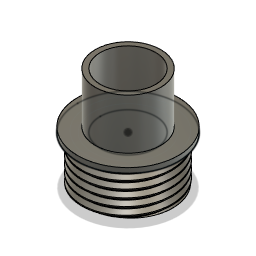
Naustok_vrch (Autodesk Fusion 360 design; units mm, degrees)
Autodesk Fusion 360 part; units mm, degrees
sketch "Sketch1" plane through (0, 0, 0) normal (0, 1, 0) x (1, 0, 0)
  circle A0 centre (0, 0) radius 9
  circle A1 centre (0, 0) radius 7
  dimension "d1" = 18
  dimension "d2" = 14
  constraint coincident A0.centre A1.centre
  measures "d1" diameter of A0
  measures "d2" diameter of A1
extrude "Extrude1" add sketch "Sketch1" along normal blind 9
thread "Thread1" "ISO Metric profile 18.0 M18x1.5 6g" major diameter 17.85 minor diameter 16.137 pitch 1.5 angle 60 modelled right hand crest width 0.2154 on face at (8.9888, 6, 0.4486) crest through (8.925, -0.375, 0)
sketch "Sketch2" plane through (0, 9, 0) normal (0, 1, 0) x (-1, 0, 0)
  spline S0 degree 3 poles (3.8907, -8.0323) (4.9021, -7.4832) (5.7974, -6.7436) (7.2383, -4.9764) (7.7758, -3.9708) (8.4256, -1.829) (8.5391, -0.7157) (8.331, 1.4708) (8.0193, 2.5236) (7.1818, 4.1155) (6.7709, 4.6996) (5.8142, 5.7398) (5.2743, 6.1931) (4.6825, 6.5707) knots 0 0 0 0 0.345232 0.345232 0.684313 0.684313 1.01724 1.01724 1.344011 1.344011 1.557735 1.557735 1.768716 1.768716 1.768716 1.768716
  arc A0 (4.6825, 6.5707) -> (-4.6825, 6.5707) centre (0, 0) ccw
  spline S1 degree 3 poles (-4.6825, 6.5707) (-5.5757, 6.0008) (-6.3478, 5.2604) (-7.58, 3.5103) (-8.0217, 2.5129) (-8.5066, 0.3852) (-8.5373, -0.7263) (-8.1712, -2.9202) (-7.7701, -3.9799) (-6.7795, -5.5785) (-6.2979, -6.1678) (-5.1891, -7.2148) (-4.5649, -7.6663) (-3.8907, -8.0323) knots 0 0 0 0 0.317853 0.317853 0.641852 0.641852 0.971995 0.971995 1.308279 1.308279 1.535261 1.535261 1.76498 1.76498 1.76498 1.76498
  arc A1 (-3.8907, -8.0323) -> (3.8907, -8.0323) centre (0, 0) ccw
  circle A2 centre (0, 0) radius 7
  circle A3 centre (0, 0) radius 10
  circle A4 centre (0, 0) radius 5.5
  dimension "d6" = 20
  constraint concentric A0 A3
  measures "d6" diameter of A3
extrude "Extrude3" add sketch "Sketch2" along normal blind 1 contours S0 A0 S1 A1 | A2 | A3
sketch "Sketch3" plane through (0, 10, 0) normal (0, 1, 0) x (-1, 0, 0)
  circle A0 centre (0, 0) radius 5.5
  circle A1 centre (0, 0) radius 10
  circle A2 centre (0, 0) radius 5.5
  circle A3 centre (0, 0) radius 6.5
  dimension "d13" = 1
  constraint coincident A0.centre A1.centre
extrude "Extrude4" add sketch "Sketch3" along normal blind 10 contours A3
